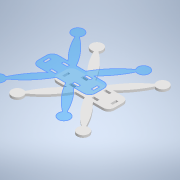
# Autodesk Inventor part: Dron
Saved by Autodesk Inventor 2022 (Build 260153000, 153)
## iProperties
Created: 2025-06-24
Part Number: Dron
Material: Типовые
Document SubType Name: Modeling
Designer: korsh524
Density: 1 g/cm^3
Appearance: По умолчанию
Author: korsh524
Autodesk Inventor part; units mm, degrees
ref_plane "YZ Plane" through (0, 0, 0) normal (1, 0, 0) x (0, 1, 0)
ref_plane "XZ Plane" through (0, 0, 0) normal (0, 1, 0) x (-1, 0, 0)
ref_plane "XY Plane" through (0, 0, 0) normal (0, 0, 1) x (1, 0, 0)
sketch "Эскиз1" plane through (0, 0, 0) normal (0, 1, 0) x (-1, 0, 0)
  line L0 (40, 17.5) -> (-40, 17.5)
  line L1 (-50, 7.5) -> (-50, -7.5)
  line L2 (-40, -17.5) -> (40, -17.5)
  line L3 (50, -7.5) -> (50, 7.5)
  line L4 (0, 0) -> (103.6754, 0) construction
  line L5 (0, 0) -> (0, -121.5896) construction
  line L6 (14.4533, -17.5) -> (50.9438, -61.6825)
  circle A0 centre (57.3118, -69.3928) radius 10
  arc A1 (53.3569, -60.2081) -> (22.4906, -17.5) centre (-76.5583, -121.5932) ccw
  line L7 (0, 0) -> (119.3987, -22.9778) construction
  arc A2 (8.22, -17.5) -> (49.04, -63.7734) centre (133.8701, 52.2004) ccw
  arc A3 (40, -17.5) -> (50, -7.5) centre (40, -7.5) ccw
  arc A4 (50, 7.5) -> (40, 17.5) centre (40, 7.5) ccw
  arc A5 (-40, 17.5) -> (-50, 7.5) centre (-40, 7.5) ccw
  arc A6 (-50, -7.5) -> (-40, -17.5) centre (-40, -7.5) ccw
  line L8 (-14.4533, -17.5) -> (-50.9438, -61.6825)
  circle A7 centre (-57.3118, -69.3928) radius 10
  arc A8 (-22.4906, -17.5) -> (-53.3569, -60.2081) centre (76.5583, -121.5932) ccw
  arc A9 (-49.04, -63.7734) -> (-8.22, -17.5) centre (-133.8701, 52.2004) ccw
  line L9 (0, 0) -> (0, 121.5896) construction
  line L10 (14.4533, 17.5) -> (50.9438, 61.6825)
  circle A10 centre (57.3118, 69.3928) radius 10
  arc A11 (22.4906, 17.5) -> (53.3569, 60.2081) centre (-76.5583, 121.5932) ccw
  arc A12 (49.04, 63.7734) -> (8.22, 17.5) centre (133.8701, -52.2004) ccw
  circle A13 centre (-57.3118, 69.3928) radius 10
  arc A14 (-53.3569, 60.2081) -> (-22.4906, 17.5) centre (76.5583, 121.5932) ccw
  line L11 (-14.4533, 17.5) -> (-50.9438, 61.6825)
  arc A15 (-8.22, 17.5) -> (-49.04, 63.7734) centre (-133.8701, -52.2004) ccw
  point P0 (50, 17.5)
  point P1 (-50, -17.5)
  point P2 (50, -17.5)
  point P3 (-22.4906, -17.5)
  point P4 (-8.22, -17.5)
  point P5 (22.4906, 17.5)
  point P6 (8.22, 17.5)
  point P7 (-8.22, 17.5)
  point P8 (-22.4906, 17.5)
  dimension "d0" = 35
  dimension "d1" = 100
  dimension "d2" = 50
  dimension "d3" = 35
  dimension "d4" = 17.5
  dimension "d5" = 80
  dimension "d6" = 20
  dimension "d7" = 10
  dimension "d8" = 10
  constraints: 36 point on circle, 30 symmetric about line, 24 end point, 16 centre point, 9 point on line, 8 tangent, 2 equal radius, 2 horizontal, 2 parallel, 1 perpendicular, 1 vertical, 10 other
  measures "d0" distance between parallel lines of L2 L0
  measures "d1" distance of point (-50, -17.5) point (50, -17.5)
  measures "d2" distance from line of L3 L4.start
  measures "d3" distance of point (50, -17.5) point (50, 17.5)
  measures "d4" distance from line of L0 L4.start
  measures "d5" distance of L4.start L6.end
  measures "d6" diameter of A0
  measures "d7" radius of A3
  measures "d8" radius of A4
extrude "Выдавливание1" add sketch "Эскиз1" along normal blind 4
sketch "Эскиз2" plane through (0, 4, 0) normal (0, 1, 0) x (1, 0, 0)
  line L0 (-25, -12.5) -> (-15, -12.5)
  line L1 (-15, -12.5) -> (-15, -8.5)
  line L2 (-15, -8.5) -> (-25, -8.5)
  line L3 (-25, -8.5) -> (-25, -12.5)
  line L4 (-50, 7.5) -> (-50, -7.5) projected
  line L5 (-40, -17.5) -> (-22.4906, -17.5) projected
  line L6 (0, 0) -> (-53.5692, 0) construction
  line L7 (0, 0) -> (0, -51.6418) construction
  line L8 (-25, 12.5) -> (-15, 12.5)
  line L9 (-15, 12.5) -> (-15, 8.5)
  line L10 (-15, 8.5) -> (-25, 8.5)
  line L11 (-25, 8.5) -> (-25, 12.5)
  line L12 (-40, 17.5) -> (-22.4906, 17.5)
  line L13 (0, 0) -> (0, 51.6418) construction
  line L14 (25, -12.5) -> (15, -12.5)
  line L15 (15, -12.5) -> (15, -8.5)
  line L16 (15, -8.5) -> (25, -8.5)
  line L17 (25, -8.5) -> (25, -12.5)
  line L18 (25, 12.5) -> (15, 12.5)
  line L19 (15, 12.5) -> (15, 8.5)
  line L20 (15, 8.5) -> (25, 8.5)
  line L21 (25, 8.5) -> (25, 12.5)
  dimension "d11" = 4
  dimension "d12" = 10
  dimension "d13" = 25
  dimension "d14" = 5
  constraints: 40 end point, 15 symmetric about line, 2 horizontal, 2 parallel, 1 perpendicular, 1 vertical
  measures "d11" distance of L2.end L0.start
  measures "d12" distance of L1.end L2.end
  measures "d13" distance between parallel lines of L4 L3
  measures "d14" distance between parallel lines of L5 L0
extrude "Выдавливание2" cut sketch "Эскиз2" against normal blind 4
sketch "Эскиз3" plane through (0, 4, 0) normal (0, 1, 0) x (1, 0, 0)
  line L0 (-40, -4.453) -> (-44, -4.453)
  line L1 (-44, -4.453) -> (-44, 5.547)
  line L2 (-44, 5.547) -> (-40, 5.547)
  line L3 (-40, 5.547) -> (-40, -4.453)
  line L4 (-50, 7.5) -> (-50, -7.5) projected
  line L5 (0, 0) -> (0, 42.0711) construction
  line L6 (40, -4.453) -> (44, -4.453)
  line L7 (44, -4.453) -> (44, 5.547)
  line L8 (44, 5.547) -> (40, 5.547)
  line L9 (40, 5.547) -> (40, -4.453)
  dimension "d17" = 10
  dimension "d18" = 4
  dimension "d19" = 10
  constraints: 18 end point, 4 symmetric about line, 2 parallel, 1 horizontal, 1 perpendicular, 1 vertical
  measures "d17" distance between parallel lines of L3 L4
  measures "d18" distance of L0.start L0.end
  measures "d19" distance of L0.end L1.end
extrude "Выдавливание3" cut sketch "Эскиз3" against normal blind 4
